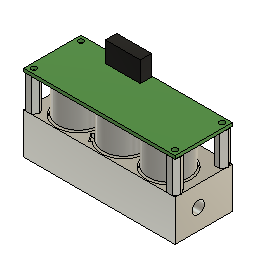
assembly-2-v10 (Autodesk Fusion 360 archive; units mm, degrees)
design "Alphasense A4 AFE 3-way v2"
Autodesk Fusion 360 part; units mm, degrees
sketch "Main Geometry" plane through (0, 0, 0) normal (0, 0, 1) x (1, 0, 0)
  line L0 (0, 0) -> (74, 0)
  line L1 (74, 0) -> (74, 28)
  line L2 (74, 28) -> (0, 28)
  line L3 (0, 28) -> (0, 0)
  circle A0 centre (2.5, 2.5) radius 1.3
  circle A1 centre (71.5, 2.5) radius 1.3
  circle A2 centre (2.5, 25.5) radius 1.3
  circle A3 centre (71.5, 25.5) radius 1.3
  circle A4 centre (15.5, 11.375) radius 10.875
  circle A5 centre (37.5, 11.375) radius 10.875
  circle A6 centre (59.5, 11.375) radius 10.875
  circle A7 centre (15.5, 11.375) radius 6.5
  circle A8 centre (37.5, 11.375) radius 6.5
  circle A9 centre (59.5, 11.375) radius 6.5
  line L4 (37.5, 11.375) -> (27.7726, 4.5638) construction
  line L5 (37.5, 11.375) -> (33.0001, 11.375) construction
  line L6 (48.0698, 15.2398) -> (50.9376, 11.144) construction
  line L7 (26.3386, 6.6117) -> (29.2065, 2.5159)
  line L8 (26.3386, 6.6117) -> (44.7358, 19.4935)
  line L9 (29.2065, 2.5159) -> (47.6036, 15.3977)
  dimension "d1" = 74
  dimension "d2" = 28
  dimension "d3" = 2.6
  dimension "d4" = 2.5
  dimension "d5" = 2.5
  dimension "d16" = 21.75
  dimension "d17" = 15.5
  dimension "d18" = 11.375
  dimension "d21" = 22
  dimension "d22" = 0
  dimension "d23" = 13
  dimension "d32" = 2.5
  dimension "d33" = 2.5
  dimension "d34" = 2.6
  dimension "d35" = 2.6
  dimension "d36" = 2.6
  dimension "d37" = 2.5
  dimension "d38" = 2.5
  dimension "d39" = 2.5
  dimension "d40" = 2.5
  dimension "d42" = 35
  dimension "d44" = 5
  dimension "d45" = 11.875
  dimension "d47" = 5
  constraint horizontal L0
  constraint vertical L1
  constraint horizontal L2
  constraint vertical L3
  constraint coincident L0.start L3.end
  constraint concentric A4 A7
  constraint coincident A5.centre A8.centre
  constraint horizontal L5
  constraint tangent A5 L6
  constraint perpendicular L4 L6
  constraint parallel L6 L7
  constraint midpoint L4.end L7
  constraint coincident A5 L8.end
  constraint perpendicular L6 L8
  constraint coincident A5 L9.end
  constraint perpendicular L6 L9
  measures "d1" distance of L0.start L0.end
  measures "d2" distance of L0.start L2.end
  measures "d3" diameter of A0
  measures "d4" distance of L3 A0.centre
  measures "d5" distance of L0 A0.centre
  measures "d16" diameter of A4
  measures "d17" distance of L3 A4.centre
  measures "d18" distance of L0 A4.centre
  measures "d23" diameter of A7
  measures "d32" distance of L2 A2.centre
  measures "d33" distance of L3 A2.centre
  measures "d34" diameter of A2
  measures "d35" diameter of A3
  measures "d36" diameter of A1
  measures "d37" distance of L2 A3.centre
  measures "d38" distance of L1 A3.centre
  measures "d39" distance of L0 A1.centre
  measures "d40" distance of L1 A1.centre
  measures "d42" angle of L4 L5
  measures "d44" distance of L6.start L6.end
  measures "d45" distance of A5.centre L4.end
  measures "d47" distance of L7.start L7.end
  measures "d95" distance of L0.start
  measures "d96" distance of L0.start
extrude "Extrude1" add sketch "Main Geometry" against normal blind 20 contours L0 L1 L2 L3 | A4 | A5 A8 L9 | A5 A8 L8 L9 | A5 L7 L8 L9 | A5 A8 L8 L9 | A5 A8 L8 | A8 L8 L9 | A8 L9 | A8 L8 | A6 | A7 | A9 makes body 1
extrude "Extrude2" cut sketch "Main Geometry" against normal blind 2 contours A4 | A5 A8 L9 | A5 A8 L8 L9 | A5 A8 L8 L9 | A5 A8 L8 | A6 bodies 1
extrude "Extrude3" cut sketch "Main Geometry" against normal blind 2 contours A5 L7 L8 L9 bodies 1
sketch "Prototype Block Side" plane through (0, 0, 0) normal (-1, 0, 0) x (0, -1, 0)
  line L0 (0, 0) -> (-28, 0)
  line L1 (-28, 0) -> (-28, -20)
  line L2 (-28, -20) -> (0, -20)
  line L3 (0, -20) -> (0, 0)
  line L4 (-11.375, 0) -> (-11.375, -20) construction
  circle A0 centre (-11.375, -10) radius 3
  dimension "d103" = 11.375
  dimension "d105" = 6
  constraint coincident L0 L4.start
  constraint coincident L2 L4.end
  constraint perpendicular L2 L4
  constraint midpoint L4 A0.centre
  measures "d103" distance of L3 L4
  measures "d105" diameter of A0
move_face "OffsetFaces1" offset -13 3 faces at (13.7098, 10.1545, 0) (39.6425, 14.6453, 0) (60.2916, 13.3919, 0) on bodies 1
extrude "Extrude4" cut sketch "Prototype Block Side" against normal up to surface (74 mm away) contours A0 bodies 1
sketch "Standoffs" plane through (0, 0, 0) normal (0, 0, 1) x (1, 0, 0)
  circle A0 centre (71.5, 25.5) radius 1.3
  circle A1 centre (71.5, 2.5) radius 1.3
  circle A2 centre (2.5, 25.5) radius 1.3
  circle A3 centre (2.5, 2.5) radius 1.3
  line L0 (1.0566, 5) -> (-0.3868, 2.5)
  line L1 (-0.3868, 2.5) -> (1.0566, 0)
  line L2 (1.0566, 0) -> (3.9434, 0)
  line L3 (3.9434, 0) -> (5.3868, 2.5)
  line L4 (5.3868, 2.5) -> (3.9434, 5)
  line L5 (3.9434, 5) -> (1.0566, 5)
  line L6 (70.0566, 5) -> (68.6132, 2.5)
  line L7 (68.6132, 2.5) -> (70.0566, 0)
  line L8 (70.0566, 0) -> (72.9434, 0)
  line L9 (72.9434, 0) -> (74.3868, 2.5)
  line L10 (74.3868, 2.5) -> (72.9434, 5)
  line L11 (72.9434, 5) -> (70.0566, 5)
  line L12 (1.0566, 28) -> (-0.3868, 25.5)
  line L13 (-0.3868, 25.5) -> (1.0566, 23)
  line L14 (1.0566, 23) -> (3.9434, 23)
  line L15 (3.9434, 23) -> (5.3868, 25.5)
  line L16 (5.3868, 25.5) -> (3.9434, 28)
  line L17 (3.9434, 28) -> (1.0566, 28)
  line L18 (70.0566, 28) -> (68.6132, 25.5)
  line L19 (68.6132, 25.5) -> (70.0566, 23)
  line L20 (70.0566, 23) -> (72.9434, 23)
  line L21 (72.9434, 23) -> (74.3868, 25.5)
  line L22 (74.3868, 25.5) -> (72.9434, 28)
  line L23 (72.9434, 28) -> (70.0566, 28)
  point P0 (2.5, 2.5)
  point P1 (71.5, 2.5)
  point P2 (2.5, 25.5)
  point P3 (71.5, 25.5)
  dimension "d71" = 2.5
  dimension "d72" = 2.5
  dimension "d73" = 2.5
  dimension "d74" = 2.5
  constraint coincident P0 A3.centre
  constraint coincident P1 A1.centre
  constraint coincident P2 A2.centre
  constraint coincident P3 A0.centre
  measures "d71" distance of P0 L5
  measures "d72" distance of P1 L11
  measures "d73" distance of P2 L17
  measures "d74" distance of P3 L23
extrude "Extrude8" add sketch "Standoffs" along normal blind 16 separate body makes body 2 at (3.7984, 25.4352, 10.6667) makes body 3 at (71.5324, 26.7996, 10.6667) makes body 4 at (3.7984, 2.4352, 10.6667) makes body 5 at (71.5324, 3.7996, 10.6667)
ref_plane "WorkPlane1" through (0, 0, 16) normal (0, 0, 1) x (1, 0, 0)
sketch "Sensor PCB" plane through (0, 0, 16) normal (0, 0, 1) x (1, 0, 0)
  circle A0 centre (2.5, 25.5) radius 1.3
  circle A1 centre (71.5, 25.5) radius 1.3
  circle A2 centre (71.5, 2.5) radius 1.3
  circle A3 centre (2.5, 2.5) radius 1.3
  line L0 (0, 28) -> (74, 28)
  line L1 (74, 28) -> (74, 0)
  line L2 (74, 0) -> (0, 0)
  line L3 (0, 0) -> (0, 28)
  circle A4 centre (15.5, 11.375) radius 10
  circle A5 centre (37.5, 11.375) radius 10
  circle A6 centre (59.5, 11.375) radius 10
  point P0 (15.5, 11.375)
  point P1 (37.5, 11.375)
  point P2 (59.5, 11.375)
  dimension "d80" = 2.5
  dimension "d81" = 2.5
  dimension "d82" = 2.5
  dimension "d83" = 2.5
  dimension "d86" = 20
  dimension "d87" = 20
  dimension "d88" = 20
  constraint horizontal L0
  constraint vertical L1
  constraint horizontal L2
  constraint vertical L3
  constraint coincident P0 A4.centre
  constraint coincident P1 A5.centre
  constraint coincident P2 A6.centre
  measures "d80" distance of A2.centre L1
  measures "d81" distance of A2.centre L2
  measures "d82" distance of A1.centre L0
  measures "d83" distance of A0.centre L3
  measures "d86" diameter of A4
  measures "d87" diameter of A5
  measures "d88" diameter of A6
extrude "Extrude9" add sketch "Sensor PCB" against normal blind 16.5 separate body contours A4 | A5 | A6 makes body 6 at (25.4503, 10.3793, 5) makes body 7 at (47.4503, 10.3793, 5) makes body 8 at (69.4503, 10.3793, 5)
fillet "Fillet1" radius 1 3 edges at (6.1767, 14.9912, -0.5) (28.1767, 14.9912, -0.5) (50.1767, 14.9912, -0.5) on bodies 6 7 8
extrude "Extrude10" add sketch "Sensor PCB" along normal blind 1.6 separate body contours L0 L1 L2 L3 | A4 | A5 | A6 makes body 9
sketch "Sketch6" plane through (0, 0, 17.6) normal (0, 0, 1) x (-1, 0, 0)
  circle A0 centre (-71.5, -25.5) radius 1.3
  circle A1 centre (-71.5, -2.5) radius 1.3
  circle A2 centre (-2.5, -2.5) radius 1.3
  circle A3 centre (-2.5, -25.5) radius 1.3
  line L0 (0, 0) -> (-74, 0)
  line L1 (-74, 0) -> (-74, -28)
  line L2 (-74, -28) -> (0, -28)
  line L3 (0, -28) -> (0, 0)
  line L4 (-18, -27.5) -> (-35, -27.5)
  line L5 (-35, -27.5) -> (-35, -22)
  line L6 (-35, -22) -> (-18, -22)
  line L7 (-18, -22) -> (-18, -27.5)
  line L8 (0, 0) -> (0, -28)
  line L9 (0, -28) -> (-74, -28)
  dimension "d95" = 17
  dimension "d96" = 5.5
  dimension "d97" = 18
  dimension "d98" = 0.5
  constraint horizontal L4
  constraint vertical L5
  constraint horizontal L6
  constraint vertical L7
  measures "d95" distance of L5.end L6.end
  measures "d96" distance of L4.end L5.end
  measures "d97" distance of L7 L8
  measures "d98" distance of L4 L9
extrude "Extrude11" add sketch "Sketch6" along normal blind 10 separate body contours L4 L5 L6 L7 makes body 10
equation "d1 = board_width"
equation "d2 = board_height"
equation "d3 = mounting_hole_diameter"
equation "gasket_inner_diameter = 13 mm"
equation "gasket_outer_diameter = 21.75 mm"
equation "gasket_height = 2 mm"
equation "hole_spacing = 22 mm" comment "Dimension verified"
equation "hole_left_offset = 15.5 mm"
equation "hole_side_offset = ( gasket_outer_diameter / 2 ) + 0.5 mm"
equation "d16 = gasket_outer_diameter"
equation "d17 = hole_left_offset"
equation "d18 = hole_side_offset"
equation "d21 = hole_spacing"
equation "d23 = gasket_inner_diameter"
equation "spacer_length = 15 mm"
equation "spacer_washer_inner_diameter = 2.5 mm"
equation "spacer_washer_outer_diameter = 4 mm"
equation "spacer_washer_thickness = 0.5 mm"
equation "mounting_hole_diameter = 2.6 mm" comment "Dimension verified"
equation "board_width = 74 mm"
equation "board_height = 28 mm"
equation "mounting_hole_edge_offset = 2.5 mm"
equation "d32 = mounting_hole_edge_offset"
equation "d33 = mounting_hole_edge_offset"
equation "d34 = mounting_hole_diameter"
equation "d35 = mounting_hole_diameter"
equation "d36 = mounting_hole_diameter"
equation "d37 = mounting_hole_edge_offset"
equation "d38 = mounting_hole_edge_offset"
equation "d39 = mounting_hole_edge_offset"
equation "d40 = mounting_hole_edge_offset"
equation "temp_sensor_angle = 35 deg"
equation "d42 = temp_sensor_angle"
equation "temp_sensor_width = 5 mm"
equation "d44 = temp_sensor_width"
equation "d45 = ( gasket_outer_diameter / 2 ) + temp_sensor_height"
equation "temp_sensor_height = 1 mm"
equation "d47 = temp_sensor_width"
equation "d48 = -block_height"
equation "d50 = -gasket_height"
equation "temp_sensor_depth = 2 mm"
equation "d53 = -temp_sensor_depth"
equation "d58 = -( block_height / 2 ) - ( channel_diameter / 2 )"
equation "d71 = standoff_diameter / 2"
equation "d72 = standoff_diameter / 2"
equation "d73 = standoff_diameter / 2"
equation "d74 = standoff_diameter / 2"
equation "standoff_length = 16 mm"
equation "standoff_diameter = 5 mm"
equation "d77 = standoff_length"
equation "d79 = standoff_length"
equation "d80 = mounting_hole_edge_offset"
equation "d81 = mounting_hole_edge_offset"
equation "d82 = mounting_hole_edge_offset"
equation "d83 = mounting_hole_edge_offset"
equation "sensor_diameter = 20 mm"
equation "sensor_height = 16.5 mm"
equation "d86 = sensor_diameter"
equation "d87 = sensor_diameter"
equation "d88 = sensor_diameter"
equation "d89 = -sensor_height"
equation "d92 = sensor_board_pcb_thickness"
equation "sensor_board_pcb_thickness = 1.6 mm"
equation "block_height = 20 mm"
equation "d103 = hole_side_offset"
equation "channel_diameter = 6 mm"
equation "d105 = channel_diameter"
named bodies: "Block", "Standoff 1", "Standoff 2", "Standoff 3", "Standoff 4", "Sensor 1", "Sensor 2", "Sensor 3", "Sensor board", "Connector and socket height"
